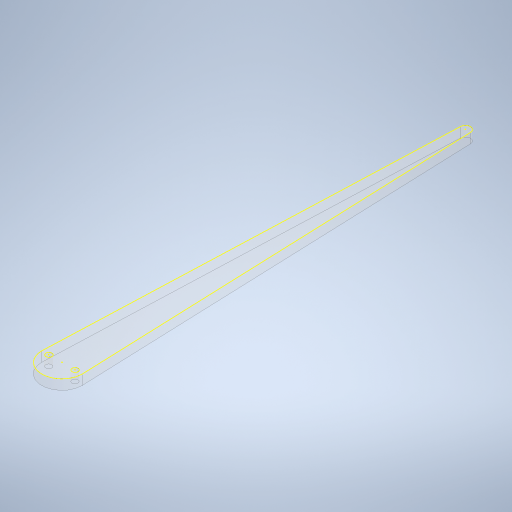
# Autodesk Inventor part: puntero
Saved by Autodesk Inventor 2024 (Build 280153000, 153)
## iProperties
Created: 2024-08-14
Part Number: puntero
Material: Polycarbonate, Clear
Document SubType Name: Modeling
Designer: David Ricaurte
Density: 1.2 g/cm^3
Appearance: Polycarbonate - Clear
Author: David Ricaurte
Autodesk Inventor part; units mm, degrees
ref_plane "YZ Plane" through (0, 0, 0) normal (1, 0, 0) x (0, 1, 0)
ref_plane "XZ Plane" through (0, 0, 0) normal (0, 1, 0) x (-1, 0, 0)
ref_plane "XY Plane" through (0, 0, 0) normal (0, 0, 1) x (1, 0, 0)
sketch "Sketch1" plane through (0, 0, 0) normal (0, 1, 0) x (-1, 0, 0)
  circle A0 centre (0, 0) radius 10
  line L0 (0, 0) -> (0, -200)
  circle A1 centre (0, -200) radius 2.5
  line L1 (0, -200) -> (-2.5, -200)
  line L2 (-2.5, -200) -> (-10, 0)
  line L3 (2.5, -200) -> (10, 0)
  circle A2 centre (0, 0) radius 6.5
  circle A3 centre (6.5, 0) radius 1.5
  circle A4 centre (-6.5, 0) radius 1.5
  dimension "d0" = 20
  dimension "d2" = 5
  dimension "d1" = 200
  dimension "d3" = 13
  dimension "d4" = 3
  dimension "d5" = 3
  constraints: 8 end point, 3 centre point, 3 coincident, 2 point on circle, 2 symmetric about line, 1 horizontal, 1 vertical, 6 other
  measures "d1" distance of L0.start L0.end
  measures "d3" diameter of A2
  measures "d4" diameter of A3
  measures "d5" diameter of A4
extrude "Extrusion1" add sketch "Sketch1" along normal blind 5 contours A2 A4 A3 | L3 A0 L2 | L3 A1 L0 A0 | A0 L0 A1 L2 | A1 L1 L0 | A1 L0 L1
sketch "Sketch2" plane through (0, 5, 0) normal (0, 1, 0) x (1, 0, 0)
  arc A0 (-10, 0) -> (10, 0) centre (0, 0) ccw projected
  line L0 (10, 0) -> (2.5, 200) projected
  arc A1 (2.5, 200) -> (-2.5, 200) centre (0, 200) ccw projected
  line L1 (-2.5, 200) -> (-10, 0) projected
  circle A2 centre (6.5, 0) radius 1.5 projected
  circle A3 centre (-6.5, 0) radius 1.5 projected
body "Solid1"
